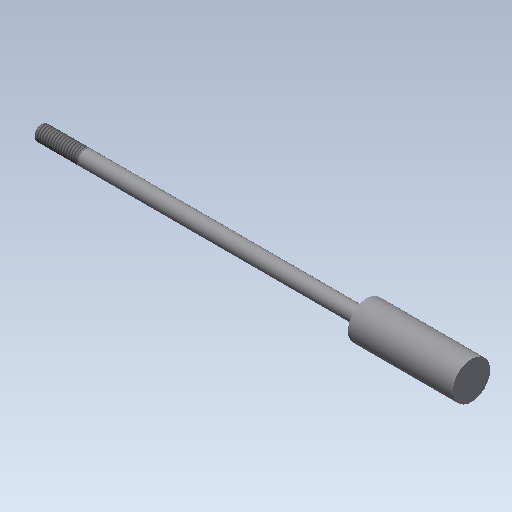
# Autodesk Inventor part: RM/8010/M/50_0_0_P
Saved by Autodesk Inventor 2020.5 (Build 245400000, 400)
## iProperties
Created: 2018-09-27
Part Number: RM/8010/M/50_0_0_P
Material: Generic
Catalog Web Link: www.cadenas.de
Description: Series RM/8000/M PART-ISO Cylinder
Vendor: IMI
Document SubType Name: Modeling
Designer: psadmin
Manufacturer: IMI
Mass: 3.29024 g
Surface Area: 21.3283 cm^2
Volume: 3.29024 cm^3
Density: 1 g/cm^3
Appearance: PSOLRGB-192-192-192
Category: PARTsolutions
Company: IMI
PSOL_IDENT_0: {$CADENAS_DATA\23d-libs\imi_precision\1_actuators\1_roundline_cylinders\parts\series_rm_8000_m_part.
PSOL_IDENT_1: prj},231 {VTYP=3D},{NB=RM/8010/M/50_0_0_P},{LINA=RM/8010/M/50_0_0_P},{NN=Series RM/8000/M PART},{DAT
PSOL_IDENT_2: E=04.09.2018 05:58:30},{GEOMDATE=13.09.2016 06:22:00},{VERSION=},{LINEID=10},{WBVAR=BS,HUB,HUBST,VAR
PSOL_IDENT_3: ,PMU,HRS,PR},{WBNUMERIC=HUB,HUBST,PMU}  {NB=RM/8010/M/50_0_0_P},{LINA=RM/8010/M/50_0_0_P},{KT=DUMMY}
PSOL_IDENT_4: ,{CNSORDERNO=RM/8010/M/50},{BS=010},{DALG=  '010' , '10' ,  '012' , '12'  ,  '016' , '16' ,   '017'
PSOL_IDENT_5: , '16' ,  '020' , '20' ,  '021' , '20'  ,  '025' , '25' ,  '026' , '25'  },{HUB=50},{HUBALG=[0:500/1
PSOL_IDENT_6: ]},{HUBST=0},{VAR=M},{VARALG=   '' , 'Standard with integral eye mounting, no variant'  , 'IU' , 'IU
PSOL_IDENT_7: - Extended piston rod'   , 'M' , 'M - Standard with integral eye mounting, no variant' ,  'MC' , 'M
PSOL_IDENT_8: C - Central rear port' ,   'MF' , 'MF - Flat rear cover' ,  'N2' , 'N2 - Non-rotating piston rod' ,
PSOL_IDENT_9: 'JM' , 'JM - Double ended piston rod'  ,  'MU' , 'MU - Extended piston rod'   },{PMU=0},{PMUALG=0},
PSOL_IDENT_10: {HRS=},{HRSALG= '' ,  'Standard (pneumatic)'  },{PR=},{PRALG= '' , 'None' , '+QM/8010/38' , 'AK - Pi
PSOL_IDENT_11: ston rod swivel' , '+QM/8010/25' , 'F - Piston rod clevis' , '+QM/8010/32' , 'UF - Piston rod eye' }
PSOL_IDENT_12: ,{AM=12},{B=12},{BA=12},{BE=M12x1.25},{BEX=12},{BF=12},{CD=4},{D=16.5},{EE=M5},{EW=7.9},{G=9.0},{KK=
PSOL_IDENT_13: M4},{KV=19},{KW=6},{KW1=2},{L=6},{L12=0},{LB=2},{MM=4},{MR=8},{PL=5.5},{KV1=7},{KV2=0},{KV4=14},{WF=
PSOL_IDENT_14: 16},{VA=1.5},{VD=1.5},{XC=64},{KKX=4.000},{KKP=0.700},{BSX=10},{SW=0},{XC2=0},{WF2=0},{BF2=0},{AD=0}
PSOL_IDENT_15: ,{AC=0},{VERS=0},{Z=0},{XYZ=0},{MOVE=0},{NEW=0}
NN: Series RM/8000/M PART
NT: ISO Cylinder
NB: RM/8010/M/50_0_0_P
NBSYN: $CNSORDERNO._$HUBST._$PMU._P
LINA: RM/8010/M/50_0_0_P
CNSORDERNO: RM/8010/M/50
BS: 10
HUB: 50
HUBST: 0
VAR: M - Standard with integral eye mounting, no variant
PMU: 0
HRS: Standard (pneumatic)
AM: 12
B: 12
BA: 12
BE: M12x1.25
BF: 12
CD: 4
D: 16.5
EE: M5
EW: 7.9
G: 9
KK: M4
KV: 19
KW: 6
KW1: 2
L: 6
L12: 0
LB: 2
MM: 4
MR: 8
PL: 5.5
WF: 16
VA: 1.5
VD: 1.5
XC: 64
SUPPLIER: IMI
ARTICLENO: RM/8010/M/50_0_0_P
BOMINFO: RM/8010/M/50_0_0_P
CREATOR: CADENAS GmbH
Title: RM/8010/M/50_0_0_P
Author: Cadenas PARTsolutions
Comments: ISO Cylinder
Autodesk Inventor part; units mm, degrees
sketch "Sketch_1" plane through (0, 0, 0) normal (0, 0, 1) x (1, 0, 0)
  line L0 (99, 0) -> (-4, 0)
  line L1 (-4, 0) -> (-4, 2)
  line L2 (-4, 2) -> (71, 2)
  line L3 (71, 2) -> (71, 5)
  line L4 (71, 5) -> (99, 5)
  line L5 (99, 5) -> (99, 0)
  line L6 (99, 0) -> (-4, 0)
  constraints: 14 end point
revolve "Revolution1" add sketch "Sketch_1" angle 360 about axis through (99, 0, 0) along (1, 0, 0)
sketch "Sketch_2" plane through (0, 0, 0) normal (0, 0, 1) x (1, 0, 0)
  line L0 (-4, 0) -> (-16, 0)
  line L1 (-16, 0) -> (-16, 1.5705)
  line L2 (-16, 1.5705) -> (-15.5705, 2)
  line L3 (-15.5705, 2) -> (-4.4295, 2)
  line L4 (-4.4295, 2) -> (-4, 1.5705)
  line L5 (-4, 1.5705) -> (-4, 0)
  line L6 (-4, 0) -> (-16, 0)
  constraints: 14 end point
revolve "Revolution2" add sketch "Sketch_2" angle 360 about axis through (-4, 0, 0) along (1, 0, 0)
thread "Thread1" size "M4x0.7" class "6g" standard "ISO Metric profile" full length
ref_plane "N_XY" through (-10, 0, 0) normal (-1, 0, 0) x (0, 0, -1)
ref_plane "N_YZ" through (-10, 0, 0) normal (0, 0, -1) x (0, -1, 0)
ref_plane "N_ZX" through (-10, 0, 0) normal (0, -1, 0) x (-1, 0, 0)
ref_plane "N2_XY" through (174, 0, 0) normal (1, 0, 0) x (0, 0, -1)
ref_plane "N2_YZ" through (174, 0, 0) normal (0, 0, -1) x (0, 1, 0)
ref_plane "N2_ZX" through (174, 0, 0) normal (0, 1, 0) x (1, 0, 0)
ref_plane "P_XY" through (0, 0, 0) normal (1, 0, 0) x (0, 0, -1)
ref_plane "P_YZ" through (0, 0, 0) normal (0, 0, -1) x (0, 1, 0)
ref_plane "P_ZX" through (0, 0, 0) normal (0, 1, 0) x (1, 0, 0)
ref_plane "dim_am1_XY" through (-16, 1.5705, 0) normal (0, 0, 1) x (1, 0, 0)
ref_plane "dim_am1_YZ" through (-16, 1.5705, 0) normal (1, 0, 0) x (0, 1, 0)
ref_plane "dim_am1_ZX" through (-16, 1.5705, 0) normal (0, 1, 0) x (0, 0, 1)
ref_plane "dim_am2_XY" through (-4, 1.5705, 0) normal (0, 0, 1) x (1, 0, 0)
ref_plane "dim_am2_YZ" through (-4, 1.5705, 0) normal (1, 0, 0) x (0, 1, 0)
ref_plane "dim_am2_ZX" through (-4, 1.5705, 0) normal (0, 1, 0) x (0, 0, 1)
ref_plane "dim_bs1_XY" through (71, 5, 0) normal (0, 0, 1) x (1, 0, 0)
ref_plane "dim_bs1_YZ" through (71, 5, 0) normal (1, 0, 0) x (0, 1, 0)
ref_plane "dim_bs1_ZX" through (71, 5, 0) normal (0, 1, 0) x (0, 0, 1)
ref_plane "dim_bs2_XY" through (71, -5, 0) normal (0, 0, 1) x (1, 0, 0)
ref_plane "dim_bs2_YZ" through (71, -5, 0) normal (1, 0, 0) x (0, 1, 0)
ref_plane "dim_bs2_ZX" through (71, -5, 0) normal (0, 1, 0) x (0, 0, 1)
ref_plane "dim_mm1_XY" through (-4, 2, 0) normal (0, 0, 1) x (1, 0, 0)
ref_plane "dim_mm1_YZ" through (-4, 2, 0) normal (1, 0, 0) x (0, 1, 0)
ref_plane "dim_mm1_ZX" through (-4, 2, 0) normal (0, 1, 0) x (0, 0, 1)
ref_plane "dim_mm2_XY" through (-4, -2, 0) normal (0, 0, 1) x (1, 0, 0)
ref_plane "dim_mm2_YZ" through (-4, -2, 0) normal (1, 0, 0) x (0, 1, 0)
ref_plane "dim_mm2_ZX" through (-4, -2, 0) normal (0, 1, 0) x (0, 0, 1)
body "Solid1"
